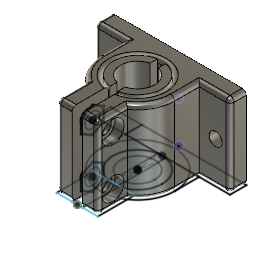
opentronsLoopHolderSmallPartWorking v6 (Autodesk Fusion 360 design; units mm, degrees)
Autodesk Fusion 360 part; units mm, degrees
sketch "main" plane through (0, 0, 0) normal (0, 0, 1) x (1, 0, 0)
  line L0 (-9, 0) -> (-9, -10)
  circle A0 centre (0, -10) radius 9
  circle A1 centre (0, -10) radius 6
  line L1 (9, -10) -> (9, -4)
  line L2 (9, -4) -> (-9, -4)
  line L3 (-9, -4) -> (-9, 0)
  line L4 (-16.5, -4) -> (16.5, -4)
  line L5 (16.5, -4) -> (16.5, 0)
  line L6 (16.5, 0) -> (-16.5, 0)
  line L7 (-16.5, 0) -> (-16.5, -4)
  line L8 (-5, -15.7024) -> (5, -15.7024)
  line L9 (5, -15.7024) -> (5, -24.7024)
  line L10 (5, -24.7024) -> (-5, -24.7024)
  line L11 (-5, -24.7024) -> (-5, -15.7024)
  line L12 (-1.25, -24.7024) -> (1.25, -24.7024)
  line L13 (1.25, -24.7024) -> (1.25, -15.7024)
  line L14 (1.25, -15.7024) -> (-1.25, -15.7024)
  line L15 (-1.25, -15.7024) -> (-1.25, -24.7024)
  point P0 (0, -4)
  point P1 (0, -4)
  point P2 (0, -24.7024)
  point P3 (0, -24.7024)
  dimension "d30" = 12
  dimension "d41" = 33
  dimension "d46" = 10
  dimension "d48" = 4
  dimension "d58" = 18
  dimension "d106" = 10
  dimension "d107" = 9
  dimension "d108" = 2.5
  constraint parallel L0 L1
  constraint tangent L0 A0
  constraint tangent A0 L1
  constraint concentric A0 A1
  constraint vertical L1
  constraint horizontal L2
  constraint vertical L3
  constraint horizontal L4
  constraint vertical L5
  constraint horizontal L6
  constraint vertical L7
  constraint midpoint L2 P1
  constraint midpoint L4 P1
  constraint vertical P1 P0
  constraint collinear L2 L4
  constraint coincident A0 L1.start
  constraint coincident A0 L0.end
  constraint vertical origin A0.centre
  constraint coincident origin L6
  constraint coincident L6 L0.start
  constraint horizontal L8
  constraint vertical L9
  constraint horizontal L10
  constraint vertical L11
  constraint midpoint L10 P3
  constraint vertical A0.centre P2
  constraint horizontal L12
  constraint vertical L13
  constraint horizontal L14
  constraint vertical L15
  constraint coincident L8 L13.end
  constraint coincident L10 L12.start
  constraint midpoint L12 P3
  measures "d30" diameter of A1
  measures "d41" distance of L5.end L6.end
  measures "d46" vertical distance of A0.centre L6.end
  measures "d48" distance of L4 L6
  measures "d58" diameter of A0
  measures "d106" distance of L9.end L10.end
  measures "d107" distance of L8.end L9.end
  measures "d108" distance of L12.start L12.end
extrude "Extrude7" add sketch "main" along normal blind 20 contours L0 A0 L2 L3 L4 L5 L6 | L0 L3 L4 L6 L7 | L0 A0 L2 L4 | A0 A1 L2 L4 L8 L11 | A0 L2 L4 | A0 A1 L8 L11 L15 | A0 L10 L11 L15 | A0 L1 L2 L4 | A0 A1 L2 L4 L8 L9 | A0 A1 L13 L15 | A0 L10 L12 L13 L15 | A0 A1 L8 L9 L13 | A0 L9 L10 L13 makes body 1
extrude "Extrude14" cut sketch "main" along normal blind 20 contours A1 L8 L14 | A0 A1 L13 L15 | A0 L10 L12 L13 L15 | A1 L8 L15 | A1 L8 L13 L14 L15 | A1 L8 L13 bodies 1
sketch "attachmentScrews" plane through (0, 0, 0) normal (0, 1, 0) x (-1, 0, 0)
  line L0 (-16.5, 0) -> (16.5, 0)
  line L1 (16.5, 0) -> (16.5, 20)
  line L2 (16.5, 20) -> (-16.5, 20)
  line L3 (-16.5, 20) -> (-16.5, 0)
  line L4 (0, 20) -> (0, 2.5)
  circle A0 centre (-13, 10) radius 1.6
  circle A1 centre (13, 10) radius 1.6
  circle A2 centre (-13, 10) radius 3.5
  circle A3 centre (13, 10) radius 3.5
  point P0 (-13, 10)
  point P1 (13, 10)
  dimension "d51" = 10
  dimension "d52" = 3.2
  dimension "d90" = 26
  dimension "d93" = 7
  constraint symmetric P0 L4 P1
  constraint coincident P0 A0.centre
  constraint symmetric L4 A0 A1
  constraint coincident P1 A1.centre
  constraint equal A2 A3
  measures "d51" vertical distance of origin A0.centre
  measures "d52" diameter of A0
  measures "d90" distance of P0 P1
  measures "d93" diameter of A2
extrude "Extrude8" cut sketch "attachmentScrews" against normal blind 4 contours A0 | A1 bodies 1
sketch "clampingNutAndScrewHole" plane through (0, 0, 0) normal (1, 0, 0) x (0, 1, 0)
  circle A0 centre (-21, 16) radius 2.7
  circle A1 centre (-21, 16) radius 1.8
  line L0 (-18.2, 17.6166) -> (-21, 19.2332)
  line L1 (-21, 19.2332) -> (-23.8, 17.6166)
  line L2 (-23.8, 17.6166) -> (-23.8, 14.3834)
  line L3 (-23.8, 14.3834) -> (-21, 12.7668)
  line L4 (-21, 12.7668) -> (-18.2, 14.3834)
  line L5 (-18.2, 14.3834) -> (-18.2, 17.6166)
  line L6 (-21, 0.7668) -> (-18.2, 2.3834)
  line L7 (-23.8, 5.6166) -> (-23.8, 2.3834)
  line L8 (-18.2, 2.3834) -> (-18.2, 5.6166)
  circle A2 centre (-21, 4) radius 1.8
  line L9 (-23.8, 2.3834) -> (-21, 0.7668)
  line L10 (-21, 7.2332) -> (-23.8, 5.6166)
  line L11 (-18.2, 5.6166) -> (-21, 7.2332)
  circle A3 centre (-21, 4) radius 2.7
  point P0 (-21, 16)
  point P1 (-21, 4)
  point P2 (0, 10)
  dimension "d100" = 5.4
  dimension "d101" = 3.6
  dimension "d102" = 21
  dimension "d111" = 0
  dimension "d112" = -12
  dimension "d113" = 5.6
  dimension "d122" = 6
  constraint concentric A0 A1
  constraint coincident P0 A0.centre
  constraint vertical L2
  constraint vertical L5
  measures "d100" diameter of A0
  measures "d101" diameter of A1
  measures "d102" horizontal distance of origin A0.centre
  measures "d113" distance of L0 L3
  measures "d122" vertical distance of P0 P2
extrude "Extrude15" cut sketch "clampingNutAndScrewHole" along normal mid plane 10 contours A1 | A2 bodies 1
extrude "Extrude16" cut sketch "clampingNutAndScrewHole" against normal blind 2.2 from surface at 5 contours A0 | A1 | A2 | A3 bodies 1
extrude "Extrude17" cut sketch "clampingNutAndScrewHole" along normal blind 2.2 from surface at -5 contours A0 | A1 | L0 L1 L2 L3 L4 L5 | L6 L7 L8 L9 L10 L11 | A2 | A3 bodies 1
fillet "Fillet5" radius 1 5 edges at (-5, -21.0929, 0) (-5, -24.7024, 10) (-5, -21.0929, 20) (5, -21.0929, 0) (5, -21.0929, 20) on bodies 1
fillet "Fillet5" radius 1 1 edges at (12.75, -4, 0) on bodies 1
fillet "Fillet7" radius 1 14 edges at (16.5, -4, 10.5) (16.5, -3.7071, 0.2929) (16.5, -1.5, 0) (12.75, -4, 20) (7.6485, -14.7434, 20) (9, -7, 20) (-9, -7, 20) (-7.6485, -14.7434, 20) (-12.75, -4, 20) (-16.5, -4, 10) (-16.5, -2, 0) (-12.75, -4, 0) (16.5, -2, 20) (-16.5, -2, 20) on bodies 1
fillet "Fillet7" radius 1 9 edges at (2.625, -24.7024, 0) (4.7071, -24.7024, 0.2929) (5, -24.7024, 10) (4.7071, -24.7024, 19.7071) (2.625, -24.7024, 20) (-2.625, -24.7024, 0) (-4.7071, -24.4095, 0.2929) (-4.7071, -24.4095, 19.7071) (-2.625, -24.7024, 20) on bodies 1
fillet "Fillet8" radius 1 6 edges at (7.6485, -14.7434, 0) (9, -6.5, 0) (-9, -6.5, 0) (-7.6485, -14.7434, 0) (-11.5083, 0, 10.5786) (14.4917, 0, 10.5786) on bodies 1
fillet "Fillet9" radius 1 1 edges at (0, -4, 20) on bodies 1
sketch "midCore" plane through (0, 0, 0) normal (0, 0, 1) x (1, 0, 0)
  circle A0 centre (0, -10) radius 5.9
  circle A1 centre (0, -10) radius 4.15
  line L0 (1, -4) -> (-1, -4)
  line L1 (-1, -4) -> (-1, -16)
  line L2 (-1, -16) -> (1, -16)
  line L3 (1, -16) -> (1, -4)
  line L4 (1, -4) -> (-1, -16) construction
  line L5 (-1, -4) -> (1, -16) construction
  point P0 (0, -10)
  point P1 (0, -10)
  dimension "d157" = 2
  dimension "d158" = 12
  dimension "d159" = 11.8
  dimension "d161" = 8.3
  constraint concentric A0 A1
  constraint horizontal L0
  constraint perpendicular L0 L1
  constraint parallel L0 L2
  constraint parallel L1 L3
  constraint coincident L4 P1
  constraint coincident L5 P1
  constraint coincident P0 A0.centre
  constraint coincident P1 P0
  measures "d157" distance of L1.end L2.end
  measures "d158" distance of L0.end L1.end
  measures "d159" diameter of A0
  measures "d161" diameter of A1
extrude "Extrude24" add sketch "midCore" along normal blind 0.4 separate body contours A1 L1 L3 | A1 L3 | A1 L1 makes body 2
extrude "Extrude22" add sketch "midCore" along normal blind 20 contours A0 A1 L3 | A0 A1 L1 bodies 2
equation "d30 = hollowCenterDiam"
equation "d42 = totalHeight"
equation "centerToBase = 10 mm"
equation "d46 = centerToBase"
equation "legThichness = 4 mm"
equation "d48 = legThichness"
equation "d53 = -legThichness"
equation "d58 = hollowCenterDiam + 2 * hollowWallThickness"
equation "hollowCenterDiam = 12 mm"
equation "nutFlatToFlatX = 5.6 mm"
equation "playX = 0.4 mm"
equation "nutHeightX = 2.2 mm"
equation "screwAndPlayHoleX = 3.2 mm"
equation "screwLen = 21.7 mm"
equation "screwHeadODiam = 5 mm"
equation "hollowWallThickness = 3 mm"
equation "totalHeight = 20 mm"
equation "nutToNutCenterDistanceX = 26 mm"
equation "d90 = nutToNutCenterDistanceX"
equation "clampingPartsHeight = totalHeight * 0.75"
equation "d93 = screwHeadODiam + 2 mm"
equation "d98 = totalHeight"
equation "d100 = screwHeadODiam + playX"
equation "d101 = screwAndPlayHoleX + playX"
equation "d113 = nutFlatToFlatX"
equation "d114 = -nutHeightX"
equation "d117 = nutHeightX"
equation "d159 = hollowCenterDiam - 0.2 mm"
equation "loopDiameter = 8 mm"
equation "d161 = loopDiameter + 0.3 mm"
equation "d162 = totalHeight"
named bodies: "penHolderUpperPart", "midCore"
